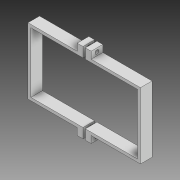
# Autodesk Inventor part: proto_clamp
Saved by Autodesk Inventor 2020 (Build 240168000, 168)
## iProperties
Created: 2021-02-05
Part Number: proto_clamp
Material: Generic
Document SubType Name: Modeling
Designer: DDeGo
Density: 1 g/cm^3
Appearance: Default
Author: DDeGo
Autodesk Inventor part; units mm, degrees
ref_plane "YZ Plane" through (0, 0, 0) normal (1, 0, 0) x (0, 1, 0)
ref_plane "XZ Plane" through (0, 0, 0) normal (0, 1, 0) x (-1, 0, 0)
ref_plane "XY Plane" through (0, 0, 0) normal (0, 0, 1) x (1, 0, 0)
sketch "Sketch6" plane through (0, 0, 0) normal (0, 0, 1) x (1, 0, 0)
  line L0 (-46, -26) -> (46, -26)
  line L1 (46, -26) -> (46, 26)
  line L2 (46, 26) -> (-46, 26)
  line L3 (-46, 26) -> (-46, -26)
  line L4 (-46, -26) -> (46, 26) construction
  line L5 (46, -26) -> (-46, 26) construction
  line L6 (-48.5, -28.5) -> (48.5, -28.5)
  line L7 (48.5, -28.5) -> (48.5, 28.5)
  line L8 (48.5, 28.5) -> (-48.5, 28.5)
  line L9 (-48.5, 28.5) -> (-48.5, -28.5)
  line L10 (-48.5, -28.5) -> (48.5, 28.5) construction
  line L11 (48.5, -28.5) -> (-48.5, 28.5) construction
  point P0 (0, 0)
  dimension "d35" = 2.5
  dimension "d36" = 2.5
  dimension "d37" = 52
  dimension "d38" = 92
  constraints: 24 end point, 4 midpoint, 4 parallel, 2 horizontal, 2 perpendicular
  measures "d35" distance between parallel lines of L7 L1
  measures "d36" distance between parallel lines of L8 L2
  measures "d37" distance between parallel lines of L0 L2
  measures "d38" distance between parallel lines of L3 L1
extrude "Extrusion6" add sketch "Sketch6" along normal blind 10
sketch "Sketch7" plane through (0, 0, 10) normal (0, 0, 1) x (1, 0, 0)
  line L0 (-1, -49.9526) -> (1, -49.9526)
  line L1 (1, -49.9526) -> (1, 49.9526)
  line L2 (1, 49.9526) -> (-1, 49.9526)
  line L3 (-1, 49.9526) -> (-1, -49.9526)
  line L4 (-1, -49.9526) -> (1, 49.9526) construction
  line L5 (1, -49.9526) -> (-1, 49.9526) construction
  point P0 (0, 0)
  dimension "d41" = 2
  constraints: 12 end point, 2 midpoint, 2 parallel, 1 horizontal, 1 perpendicular
  measures "d41" distance of L1.end L2.end
extrude "Extrusion7" cut sketch "Sketch7" against normal through all
sketch "Sketch8" plane through (0, 0, 10) normal (0, 0, 1) x (1, 0, 0)
  line L0 (-1, 28.5) -> (-48.5, 28.5) projected
  line L1 (-1, 28.5) -> (-6, 28.5)
  line L2 (-6, 28.5) -> (-6, 34.5)
  line L3 (-6, 34.5) -> (-1, 34.5)
  line L4 (-1, 34.5) -> (-1, 28.5)
  line L5 (48.5, 28.5) -> (1, 28.5) projected
  line L6 (1, 28.5) -> (6, 28.5)
  line L7 (6, 28.5) -> (6, 34.5)
  line L8 (6, 34.5) -> (1, 34.5)
  line L9 (1, 34.5) -> (1, 28.5)
  line L10 (-1, -26) -> (-1, -28.5) projected
  line L11 (-1, -28.5) -> (-6, -28.5)
  line L12 (-6, -28.5) -> (-6, -34.5)
  line L13 (-6, -34.5) -> (-1, -34.5)
  line L14 (-1, -34.5) -> (-1, -28.5)
  line L15 (1, -28.5) -> (48.5, -28.5) projected
  line L16 (1, -28.5) -> (6, -28.5)
  line L17 (6, -28.5) -> (6, -34.5)
  line L18 (6, -34.5) -> (1, -34.5)
  line L19 (1, -34.5) -> (1, -28.5)
  point P0 (0, 0)
  dimension "d44" = 5
  dimension "d45" = 6
  constraints: 32 end point, 8 parallel, 6 equal length, 4 horizontal, 4 perpendicular, 1 point on line
  measures "d44" distance of L17.end L18.end
  measures "d45" distance of L16.end L17.end
extrude "Extrusion8" add sketch "Sketch8" against normal up to surface (10 mm away)
sketch "Sketch9" plane through (-6, -34.5, 10) normal (-1, 0, 0) x (0, 0, 1)
  line L0 (0, 69) -> (-10, 69) construction
  line L1 (-5, 69) -> (-5, 63) construction
  line L2 (0, 63) -> (-10, 63) construction
  line L3 (-10, 6) -> (0, 6) construction
  line L4 (-5, 6) -> (-5, 0) construction
  line L5 (0, 0) -> (-10, 0) construction
  circle A0 centre (-5, 3) radius 1.65
  circle A1 centre (-5, 66) radius 1.65
  point P0 (-10, 34.5)
  dimension "d48" = 3.3
  constraints: 6 midpoint, 4 end point, 2 centre point, 1 equal radius
  measures "d48" diameter of A0
extrude "Extrusion9" cut sketch "Sketch9" against normal through all
equation "\"d36\" = d35"
body "Solid2"
